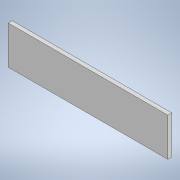
# Autodesk Inventor part: mini-JLT_placeholder
Saved by Autodesk Inventor 2020.2 (Build 242310000, 310)
## iProperties
Created: 2020-10-15
Part Number: mini-JLT_placeholder
Material: Generic
Document SubType Name: Modeling
Designer: Krishna Makhija
Density: 1 g/cm^3
Appearance: Default
Author: Krishna Makhija
Autodesk Inventor part; units mm, degrees
ref_plane "YZ Plane" through (0, 0, 0) normal (1, 0, 0) x (0, 1, 0)
ref_plane "XZ Plane" through (0, 0, 0) normal (0, 1, 0) x (-1, 0, 0)
ref_plane "XY Plane" through (0, 0, 0) normal (0, 0, 1) x (1, 0, 0)
sketch "Sketch1" plane through (0, 0, 0) normal (0, 0, 1) x (1, 0, 0)
  line L0 (63.4971, -15.244) -> (-63.4971, -15.244)
  line L1 (-63.4971, -15.244) -> (-63.4971, 15.244)
  line L2 (-63.4971, 15.244) -> (63.4971, 15.244)
  line L3 (63.4971, 15.244) -> (63.4971, -15.244)
  line L4 (63.4971, -15.244) -> (-63.4971, 15.244) construction
  line L5 (-63.4971, -15.244) -> (63.4971, 15.244) construction
  point P0 (0, 0)
  constraints: 12 end point, 2 midpoint, 2 parallel, 1 horizontal, 1 perpendicular
extrude "Extrusion1" add sketch "Sketch1" along normal blind 3.175
body "Solid1"
